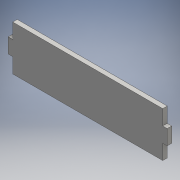
# Autodesk Inventor part: support
Saved by Autodesk Inventor 2016 (Build 200138000, 138)
## iProperties
Created: 2019-02-01
Part Number: support
Material: Generic
Document SubType Name: Modeling
Designer: LinJie
Density: 1 g/cm^3
Appearance: Default
Author: LinJie
Autodesk Inventor part; units mm, degrees
ref_plane "YZ Plane" through (0, 0, 0) normal (1, 0, 0) x (0, 1, 0)
ref_plane "XZ Plane" through (0, 0, 0) normal (0, 1, 0) x (-1, 0, 0)
ref_plane "XY Plane" through (0, 0, 0) normal (0, 0, 1) x (1, 0, 0)
sketch "Sketch1" plane through (0, 0, 0) normal (0, 1, 0) x (-1, 0, 0)
  line L0 (50, 15) -> (-50, 15)
  line L1 (-50, 15) -> (-50, -15)
  line L2 (-50, -15) -> (50, -15)
  line L3 (50, -15) -> (50, 15)
  line L4 (50, 15) -> (-50, -15) construction
  line L5 (-50, 15) -> (50, -15) construction
  line L6 (-50, -5) -> (-53, -5)
  line L7 (-53, -5) -> (-53, 5)
  line L8 (-53, 5) -> (-50, 5)
  line L9 (-50, 5) -> (-50, -5)
  line L10 (50, -5) -> (53, -5)
  line L11 (53, -5) -> (53, 5)
  line L12 (53, 5) -> (50, 5)
  line L13 (50, 5) -> (50, -5)
  point P0 (0, 0)
  point P1 (50, 0)
  dimension "d0" = 100
  dimension "d1" = 30
  dimension "d2" = 3
  dimension "d3" = 10
  dimension "d4" = 3
  constraints: 28 end point, 6 parallel, 4 midpoint, 4 point on line, 3 horizontal, 3 perpendicular
  measures "d0" distance of L2.end L1.end
  measures "d1" distance of L1.end L0.end
  measures "d2" distance of L6.start L6.end
  measures "d3" distance of L6.end L7.end
  measures "d4" distance of L10.start L10.end
extrude "Extrusion1" add sketch "Sketch1" along normal blind 3
body "Solid1"
